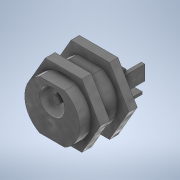
# Autodesk Inventor part: Jack
Saved by Autodesk Inventor 2020.5 (Build 245400000, 400)
## iProperties
Created: 2022-12-15
Part Number: Jack
Material: Generic
Document SubType Name: Modeling
Designer: aivel
Density: 1 g/cm^3
Appearance: Fine Textured - Black
Author: aivel
Autodesk Inventor part; units mm, degrees
ref_plane "YZ Plane" through (0, 0, 0) normal (1, 0, 0) x (0, 1, 0)
ref_plane "XZ Plane" through (0, 0, 0) normal (0, 1, 0) x (-1, 0, 0)
ref_plane "XY Plane" through (0, 0, 0) normal (0, 0, 1) x (1, 0, 0)
sketch "Sketch1" plane through (0, 0, 0) normal (0, 0, 1) x (1, 0, 0)
  line L0 (4.5611, 7.9) -> (9.1221, 0)
  line L1 (9.1221, 0) -> (4.5611, -7.9)
  line L2 (4.5611, -7.9) -> (-4.5611, -7.9)
  line L3 (-4.5611, -7.9) -> (-9.1221, 0)
  line L4 (-9.1221, 0) -> (-4.5611, 7.9)
  line L5 (-4.5611, 7.9) -> (4.5611, 7.9)
  circle A0 centre (0, 2) radius 1
  circle A1 centre (0, 2) radius 3
  line L6 (4.3301, 7.5) -> (8.6603, 0)
  line L7 (8.6603, 0) -> (4.3301, -7.5)
  line L8 (4.3301, -7.5) -> (-4.3301, -7.5)
  line L9 (-4.3301, -7.5) -> (-8.6603, 0)
  line L10 (-8.6603, 0) -> (-4.3301, 7.5)
  line L11 (-4.3301, 7.5) -> (4.3301, 7.5)
  line L12 (4.1, 3.75) -> (4.1, 0.25)
  line L13 (4.1, 0.25) -> (4.9, 0.25)
  line L14 (4.9, 0.25) -> (4.9, 3.75)
  line L15 (4.9, 3.75) -> (4.1, 3.75)
  line L16 (0.38, -3.1) -> (3.38, -3.1)
  line L17 (3.38, -3.1) -> (3.38, -3.7)
  line L18 (3.38, -3.7) -> (0.38, -3.7)
  line L19 (0.38, -3.7) -> (0.38, -3.1)
  line L20 (-3.02, -0.95) -> (-0.02, -0.95)
  line L21 (-0.02, -0.95) -> (-0.02, -1.55)
  line L22 (-0.02, -1.55) -> (-3.02, -1.55)
  line L23 (-3.02, -1.55) -> (-3.02, -0.95)
  line L24 (-4.5, 4.5) -> (4.5, 4.5)
  line L25 (4.5, 4.5) -> (4.5, -4.5)
  line L26 (4.5, -4.5) -> (-4.5, -4.5)
  line L27 (-4.5, -4.5) -> (-4.5, 4.5)
  circle A2 centre (0, 0) radius 6.5
  line L28 (-5.8, -5.8) -> (5.8, -5.8)
  line L29 (5.8, -5.8) -> (5.8, 5.8)
  line L30 (5.8, 5.8) -> (-5.8, 5.8)
  line L31 (-5.8, 5.8) -> (-5.8, -5.8)
  point P0 (-2.9343, -5.8)
  point P1 (2.9343, -5.8)
  point P2 (2.9343, 5.8)
  point P3 (-2.9343, 5.8)
  point P4 (5.8, -5.7541)
  point P5 (5.8, 5.7541)
  point P6 (5.7735, 5.8)
  point P7 (-5.7735, 5.8)
  point P8 (-5.8, 5.7541)
  point P9 (-5.8, -5.7541)
  point P10 (-5.7735, -5.8)
  point P11 (5.7735, -5.8)
  constraints: 64 end point, 10 parallel, 5 perpendicular, 3 centre point, 3 horizontal, 2 coincident
extrude "Extrusion4" add sketch "Sketch1" against normal blind 9 contours A2 L29 L28 L31 L30 | A2 L29 | L31 A2 | A1 L24 L25 L15 L12 L13 L26 L27 L20 L23 L22 L21 | L21 L22 L23 L20 A1 | L25 L13 L12 L15 | L15 L14 L13 L25 | L16 L17 L18 L19
extrude "Extrusion5" add sketch "Sketch1" against normal blind 2 from surface at -9 contours L0 L30 L6 L11 L10 L4 L5 | L0 L29 L6 L30 | L0 L1 L29 L7 L6 | L30 A2 L10 L11 L6 | L6 L29 A2 L30 | L30 L10 L31 L4 | L6 L7 L29 A2 | L30 A2 | A2 L29 L28 L31 L30 | L31 L10 L9 L3 L4 | L30 A2 L31 L10 | L1 L28 L7 L29 | A2 L29 | L31 A2 L9 L10 | L1 L2 L3 L28 L9 L8 L7 | L7 L28 A2 L29 | L31 A2 | L31 L9 L28 L3 | L7 L8 L9 L28 A2 | A2 L28 | A2 L28 L9 L31 | A0 | A1 L21 L20 L24 | A1 L24 L25 L15 L12 L13 L26 L27 L20 L23 L22 L21 | L24 A1 | L21 L22 L23 L20 A1 | A1 L20 L21 | L25 L13 L12 L15 | L15 L14 L13 L25 | L16 L17 L18 L19
extrude "Extrusion6" add sketch "Sketch1" against normal blind 2 from surface at -11 contours A0 | A1 L21 L20 L24 | A1 L24 L25 L15 L12 L13 L26 L27 L20 L23 L22 L21 | L21 L22 L23 L20 A1 | A1 L20 L21 | L25 L13 L12 L15 | L16 L17 L18 L19
extrude "Extrusion7" add sketch "Sketch1" against normal blind 4.9 from surface at -13 contours L21 L22 L23 L20 A1 | A1 L20 L21 | L16 L17 L18 L19
extrude "Extrusion8" add sketch "Sketch1" against normal blind 6 from surface at -11 contours L25 L13 L12 L15 | L15 L14 L13 L25
extrude "Extrusion9" add sketch "Sketch1" along normal blind 6.3 from surface at -9 contours L30 A2 L10 L11 L6 | L6 L29 A2 L30 | L6 L7 L29 A2 | L30 A2 L31 L10 | L31 A2 L9 L10 | L7 L28 A2 L29 | L7 L8 L9 L28 A2 | A2 L28 L9 L31
extrude "Extrusion10" cut sketch "Sketch1" along normal blind 4 from surface at -9 contours L30 A2 L10 L11 L6 | L6 L29 A2 L30 | L6 L7 L29 A2 | L30 A2 L31 L10 | L31 A2 L9 L10 | L7 L28 A2 L29 | L7 L8 L9 L28 A2 | A2 L28 L9 L31
extrude "Extrusion11" add sketch "Sketch1" along normal blind 8 from surface at -9 contours A0
body "Solid2"
